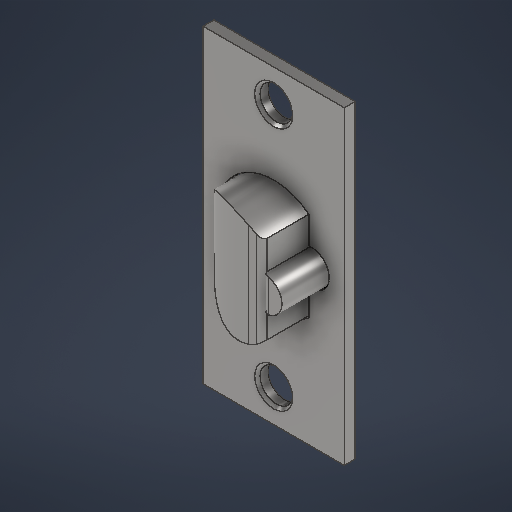
# Autodesk Inventor part: LOK-58 CERRADURA PICAPORTE (PASADOR)
Saved by Autodesk Inventor 2025 (Build 290162000, 162)
## iProperties
Created: 2026-02-18
Part Number: LOK-58 CERRADURA PICAPORTE (PASADOR)
Material: Acero inoxidable
Document SubType Name: Modeling
Designer: ROLANDO
Density: 8 g/cm^3
Appearance: Semipulido
Author: ROLANDO
Autodesk Inventor part; units mm, degrees
ref_plane "YZ Plane" through (0, 0, 0) normal (1, 0, 0) x (0, 1, 0)
sketch "Boceto1" plane through (-57, 0, 0) normal (0, 0, 1) x (1, 0, 0)
  line L0 (-13, 28.5) -> (13, 28.5)
  line L1 (13, 28.5) -> (13, -28.5)
  line L2 (13, -28.5) -> (-13, -28.5)
  line L3 (-13, -28.5) -> (-13, 28.5)
  line L4 (-13, 28.5) -> (13, -28.5) construction
  line L5 (13, 28.5) -> (-13, -28.5) construction
  circle A0 centre (0, 0) radius 10.5 projected
  line L6 (6.5, -8.2462) -> (6.5, -3.1943)
  line L7 (6.5, 8.2462) -> (6.5, 3.1943)
  line L8 (10.2924, 0) -> (-1.6343, 0) construction
  arc A1 (6.5, -3.1943) -> (6.5, 3.1943) centre (7, 0) ccw
  arc A2 (6.5, -8.2462) -> (6.5, 8.2462) centre (0, 0) ccw construction
  point P0 (5.5, 0)
  dimension "d27" = 13
  dimension "d68" = 6.5
  dimension "d69" = 3.2332
  dimension "d72" = 0.5
  dimension "d105" = 28.5
  dimension "d106" = 26
  dimension "d107" = 57
  constraints: 18 end point, 4 point on circle, 2 centre point, 2 horizontal, 2 midpoint, 2 parallel, 1 collinear, 1 perpendicular, 1 point on line, 1 vertical
  measures "d27" distance from line of A0.centre L1
  measures "d68" distance from line of point (0, 0) L6
  measures "d69" radius of A1
  measures "d72" distance from line of L6 A1.centre
  measures "d105" distance from line of point (0, 0) L0
  measures "d106" distance of L1.end L2.end
  measures "d107" distance of L0.end L1.end
extrude "Extrusión1" add sketch "Boceto1" along normal blind 2 contours L0 L1 L2 L3 | A0 L6 A1 L7 picked at (7.0604, -6.0073)
ref_plane "Plano de trabajo1" through (-57, 0, 0) normal (0, 0, -1) x (-1, 0, 0)
sketch "Boceto2" plane through (-57, 0, 0) normal (0, 0, 1) x (1, 0, 0)
  line L0 (6.5, 2.9943) -> (6.5, -2.9943)
  arc A0 (6.5, -2.9943) -> (6.5, 2.9943) centre (7, 0) ccw
  line L1 (6.3, 8.0853) -> (6.3, -8.0853)
  arc A1 (6.3, 8.0853) -> (6.3, -8.0853) centre (0, 0) ccw
  point P0 (6.5, 0)
  dimension "d41" = 3.0357
  dimension "d42" = 0.5
  dimension "d43" = 0.2
  dimension "d111" = 20.5
  constraints: 4 end point, 4 point on circle, 2 centre point, 2 vertical, 1 midpoint
  measures "d41" radius of A0
  measures "d42" distance from line of L0 A0.centre
  measures "d43" distance between parallel lines of L1 L0
  measures "d111" diameter of A1
extrude "Extrusión2" add sketch "Boceto2" along normal blind 10.5
ref_plane "Plano de trabajo2" through (-70, -28.5, 0) normal (0, -1, 0) x (1, 0, 0)
sketch "Boceto3" plane through (-57, -28.5, 0) normal (0, -1, 0) x (1, 0, 0)
  line L0 (6.3, 2) -> (-10.25, 2)
  arc A0 (6.3, 10.5) -> (-10.25, 2) centre (5.0652, -7.4576) ccw
  line L1 (6.3, 2) -> (6.3, 10.5)
  line L2 (6.3, 10.5) -> (-10.25, 10.5)
  line L3 (-10.25, 10.5) -> (-10.25, 2)
  point P0 (57, 0)
  point P1 (3.8303, 10.5)
  dimension "d110" = 18
  constraints: 8 end point, 2 point on circle, 1 centre point, 1 horizontal, 1 perpendicular, 1 vertical
  measures "d110" radius of A0
extrude "Extrusión3" cut sketch "Boceto3" against normal up to surface (57 mm away) contours L3 L2 A0
fillet "Empalme3" radius 1 2 edges at (-50.7, 0, 10.5) (-50.5, 0, 10.5)
sketch "Boceto12" plane through (-57, 0, 2) normal (0, 0, 1) x (1, 0, 0)
  circle A0 centre (0, 22.5) radius 3
  line L0 (13, 28.5) -> (-13, 28.5) projected
  circle A1 centre (0, -22.5) radius 3
  line L1 (-13, -28.5) -> (13, -28.5) projected
  line L2 (13, -28.5) -> (13, 28.5) projected
  line L3 (-13, 28.5) -> (-13, -28.5) projected
  point P0 (57, 0)
  dimension "d114" = 6
  dimension "d115" = 6
  dimension "d116" = 6
  dimension "d117" = 6
  dimension "d118" = 13
  dimension "d119" = 13
  dimension "d120" = 13
  dimension "d121" = 13
  dimension "d122" = 45
  constraints: 2 centre point
  measures "d114" diameter of A0
  measures "d115" distance from line of L0 A0.centre
  measures "d116" diameter of A1
  measures "d117" distance from line of L1 A1.centre
  measures "d118" distance from line of L2 A1.centre
  measures "d119" distance from line of L2 A0.centre
  measures "d120" distance from line of L3 A1.centre
  measures "d121" distance from line of L3 A0.centre
  measures "d122" distance of A1.centre A0.centre
hole "Agujero2" at (-57, 22.5, 2) at (-57, -22.5, 2) direction (0, 0, -1) diameter 6 depth 2 countersink diameter 7 countersink angle 90
